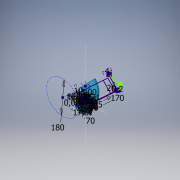
# Autodesk Inventor part: DriveChainEnclosure V3
Saved by Autodesk Inventor 2019.1 (Build 231200000, 200)
## iProperties
Created: 2018-07-04
Part Number: DriveChainEnclosure V3
Material: Generisch
Document SubType Name: Modeling
Designer: JochenAlt
Density: 1 g/cm^3
Appearance: Vorgabe
Mass: 189.121 g
Surface Area: 1542.72 cm^2
Volume: 189.121 cm^3
Author: JochenAlt
Autodesk Inventor part; units mm, degrees
ref_plane "YZ Plane" through (0, 0, 0) normal (1, 0, 0) x (0, 1, 0)
sketch "Enclosure" plane through (0, 0, 0) normal (0, 1, 0) x (-1, 0, 0)
  line L0 (35, 0) -> (-35, 0) construction
  circle A0 centre (26.215, 0) radius 8.785 construction
  circle A1 centre (-26.215, 0) radius 8.785 construction
  circle A2 centre (125, 0) radius 90 construction
  line L1 (0, -158.2918) -> (0, 319.751) construction
  line L2 (33.1583, 39.5344) -> (33.1583, 50.6343)
  line L3 (50.6835, 69.3012) -> (48.9666, 70.9023)
  line L4 (35, 0) -> (125, 0) construction
  line L5 (33.1583, 50.6343) -> (32.1474, 52.6444)
  arc A3 (33.1583, 50.6343) -> (33.3815, 50.747) centre (0, 116.5644) ccw
  line L6 (30.6583, 49.4353) -> (30.6583, 51.917)
  line L7 (33.3815, 50.747) -> (32.2506, 52.9767)
  line L8 (30.6583, 39.5344) -> (30.6583, 49.4353)
  line L9 (32.035, 52.8678) -> (30.9118, 55.1012)
  arc A4 (16, 52.2253) -> (31.759, 58.3675) centre (0, 116.5644) ccw
  arc A5 (0, 47.7657) -> (30.9118, 55.1012) centre (0, 116.5644) ccw
  arc A6 (-30.9118, 55.1012) -> (0, 47.7657) centre (0, 116.5644) ccw
  line L10 (33.7963, 54.6342) -> (31.759, 58.3675)
  line L11 (18.3935, -4) -> (-18.3935, -4) construction
  line L12 (18.3935, 4) -> (-18.3935, 4) construction
  line L13 (30.4083, 49.3217) -> (30.4083, 52.0753)
  arc A7 (16, 47.0842) -> (30.4083, 52.0753) centre (0, 116.5644) ccw
  line L14 (-30.6583, 39.5344) -> (-30.6583, 49.4353)
  line L15 (-30.6583, 49.4353) -> (-30.6583, 51.917)
  line L16 (-33.1583, 50.6343) -> (-32.1474, 52.6444)
  line L17 (-32.035, 52.8678) -> (-30.9118, 55.1012)
  line L18 (-30.4083, 49.3217) -> (-30.4083, 52.0753)
  arc A8 (-31.759, 58.3675) -> (-16, 52.2253) centre (0, 116.5644) ccw
  line L19 (-16, 50.1663) -> (-16, 52.2253)
  arc A9 (-30.8936, 55.6522) -> (-16, 50.1663) centre (0, 116.5644) ccw
  arc A10 (16, 50.1663) -> (30.8936, 55.6522) centre (0, 116.5644) ccw
  line L20 (-16, 49.6521) -> (-16, 47.0842)
  line L21 (-31.759, 58.3675) -> (31.759, 58.3675) construction
  arc A11 (-33.3815, 50.747) -> (-33.1583, 50.6343) centre (0, 116.5644) ccw
  arc A12 (-32.035, 52.8678) -> (-30.4083, 52.0753) centre (0, 116.5644) ccw
  line L22 (-33.3815, 50.747) -> (-32.2506, 52.9767)
  arc A13 (30.4083, 52.0753) -> (32.035, 52.8678) centre (0, 116.5644) ccw
  line L23 (32.2506, 52.9767) -> (30.8936, 55.6522)
  line L24 (16, 47.0842) -> (16, 49.6521)
  line L25 (16, 50.1663) -> (16, 52.2253)
  arc A14 (30.4083, 49.3217) -> (33.1583, 50.6343) centre (0, 116.5644) ccw
  arc A15 (0, 42.7657) -> (30.4083, 49.3217) centre (0, 116.5644) ccw
  arc A16 (0, 45.2657) -> (16, 47.0842) centre (0, 116.5644) ccw
  arc A17 (-30.6583, 49.4353) -> (-30.4083, 49.3217) centre (0, 116.5644) ccw
  arc A18 (-30.4083, 49.3217) -> (0, 42.7657) centre (0, 116.5644) ccw
  arc A19 (-30.4083, 52.0753) -> (0, 45.2657) centre (0, 116.5644) ccw
  line L26 (-30.8936, 55.6522) -> (-32.2506, 52.9767)
  line L27 (-32.2506, 52.9767) -> (-39.4034, 59.6467)
  line L28 (-31.759, 58.3675) -> (-33.7731, 54.3964)
  line L29 (32.2506, 52.9767) -> (33.7963, 54.6342)
  line L30 (33.7963, 54.6342) -> (48.9666, 70.9023)
  line L31 (33.3815, 50.747) -> (50.6835, 69.3012)
  line L32 (50.6835, 69.3012) -> (48.9666, 70.9023)
  line L33 (59.1782, 61.3799) -> (125, 0) construction
  line L34 (125, 0) -> (0, 116.5644) construction
  arc A20 (32.035, 52.8678) -> (32.2506, 52.9767) centre (0, 116.5644) ccw
  line L35 (0, 42.7657) -> (0, 45.2657)
  line L36 (0, 47.7657) -> (0, 45.2657)
  arc A21 (-32.2506, 52.9767) -> (-32.035, 52.8678) centre (0, 116.5644) ccw
  line L37 (16, 49.6521) -> (16, 50.1663)
  line L38 (-16, 49.6521) -> (-16, 50.1663)
  line L39 (-178.3606, 189.2264) -> (-131.6437, 239.3241) construction
  arc A22 (-33.1583, 50.6343) -> (-30.6583, 49.4353) centre (0, 116.5644) ccw
  line L40 (-41.1083, 57.8183) -> (-39.4034, 59.6467)
  line L41 (-39.4034, 59.6467) -> (-138.1361, 151.7165)
  arc A23 (-33.1583, 39.5344) -> (-35.3024, 49.664) centre (-58.1583, 39.5344) ccw
  line L42 (-33.1583, 50.6343) -> (-35.3024, 49.664)
  line L43 (-33.3815, 50.747) -> (-35.382, 49.8417)
  arc A24 (-35.382, 49.8417) -> (-41.1083, 57.8183) centre (-58.1583, 39.5344) ccw
  line L44 (42.1466, 63.5888) -> (0.4936, 102.4309)
  line L45 (0.4936, 102.4309) -> (-39.4034, 59.6467)
  line L46 (0.4936, 102.4309) -> (-123.8366, 218.3706)
  arc A25 (-35.3024, 49.664) -> (-35.382, 49.8417) centre (-58.1583, 39.5344) ccw
  line L47 (-138.1361, 151.7165) -> (-139.8411, 149.8881)
  line L48 (-123.8366, 218.3706) -> (-163.7335, 175.5864)
  line L49 (-138.1361, 151.7165) -> (-178.3606, 189.2264)
  line L50 (-41.1083, 57.8183) -> (-139.8411, 149.8881)
  line L51 (-180.0655, 187.398) -> (-139.8411, 149.8881)
  line L52 (-33.1583, 39.5344) -> (-30.6583, 39.5344) construction
  line L53 (-26, 14.7657) -> (-24.5156, 16.7773) construction
  spline S0 degree 4 poles (-33.1583, 39.5344) (-33.1583, 29.5735) (-31.4502, 7.8306) (0, 7.8211) (31.4502, 7.8306) (33.1583, 29.5735) (33.1583, 39.5344) knots 0 0 0 0 0 0.375 0.625 1 1 1 1 1
  line L54 (24.5156, 16.7773) -> (26, 14.7657) construction
  spline S1 degree 4 poles (-30.6583, 39.5344) (-30.6583, 30.3799) (-29.8014, 10.1412) (0, 10.5514) (29.8014, 10.1412) (30.6583, 30.3799) (30.6583, 39.5344) knots 0 0 0 0 0 0.375 0.625 1 1 1 1 1
  line L55 (-138.1361, 151.7165) -> (-98.2392, 194.5006)
  line L56 (-178.3606, 189.2264) -> (-180.0655, 187.398)
  spline S2 degree 3 poles (-180.0655, 187.398) (-233.1049, 241.3232) (-158.3203, 210.7169) (-131.6437, 239.3241) knots 0 0 0 0 1 1 1 1
  line L57 (-131.6437, 239.3241) -> (-128.7183, 236.5961)
  line L58 (-128.7183, 236.5961) -> (-175.4351, 186.4984)
  arc A26 (-30.6583, 48.886) -> (30.6583, 48.886) centre (0, 116.5644) ccw
  arc A27 (-32.1474, 52.6444) -> (-30.6583, 51.917) centre (0, 116.5644) ccw
  arc A28 (30.6583, 51.917) -> (32.1474, 52.6444) centre (0, 116.5644) ccw
  line L59 (-175.2987, 186.6446) -> (-178.2242, 189.3726)
  line L60 (-178.2242, 189.3726) -> (-178.3606, 189.2264)
  point P0 (0, 0)
  point P1 (0, 5)
  point P2 (0, 58.3675)
  point P3 (0, 8)
  point P4 (0, 22.5)
  point P5 (0, 10.5)
  point P6 (-191.4493, 221.539)
  point P7 (0, 50)
  dimension "d31" = 70
  dimension "d32" = 17.57
  dimension "d42" = 180
  dimension "d106" = 0
  dimension "d672" = 0.25
  dimension "d1173" = 2.5
  dimension "d1238" = 8
  dimension "d1249" = 0.25
  dimension "d1648" = 1
  dimension "d1792" = 32
  dimension "d1795" = 2
  dimension "d1872" = 10
  dimension "d2014" = 10
  dimension "d2069" = 135
  dimension "d2070" = 20
  dimension "d2071" = 2.5
  dimension "d2072" = 71
  dimension "d2075" = 170
  dimension "d2076" = 26
  dimension "d2077" = 28
  dimension "d2079" = 8
  dimension "d2080" = 14.5
  dimension "d2081" = 2.5
  dimension "d2082" = 3
  dimension "d2252" = 0.5
  dimension "d2255" = 0.25
  dimension "d2303" = 0.5
  dimension "d2367" = 2.5
  dimension "d2369" = 0.2
  dimension "d2370" = 4
  dimension "d2395" = 43
  dimension "d2396" = 50
  dimension "d2397" = 2.5
  dimension "d2398" = 25
  constraints: 124 end point, 79 point on circle, 29 centre point, 22 point on line, 16 perpendicular, 14 coincident, 12 vertical, 11 collinear, 9 parallel, 8 line through centre, 6 equal length, 5 horizontal alignment, 4 horizontal, 3 concentric, 3 equal radius, 2 midpoint, 2 tangent, 25 other
  measures "d31" distance of L0.end L0.start
  measures "d32" diameter of A0
  measures "d42" diameter of A2
  measures "d106" distance between parallel lines of L4 L0
  measures "d672" distance of L7.start L2.end
  measures "d1173" radial gap between concentric circles of A4 A5
  measures "d1238" distance between parallel lines of L11 L12
  measures "d1249" distance between parallel lines of L6 L13
  measures "d1648" distance from line of L12 point (0, 5)
  measures "d1792" distance between parallel lines of L25 L19
  measures "d1795" distance between parallel lines of L28 L26
  measures "d1872" distance from line of A3.centre L40
  measures "d2014" distance between parallel lines of L34 L44
  measures "d2069" distance between parallel lines of L45 L47
  measures "d2070" distance between parallel lines of L48 L39
  measures "d2071" distance of L40.start L27.end
  measures "d2072" distance between parallel lines of L50 L34
  measures "d2075" distance between parallel lines of L48 L45
  measures "d2077" vertical distance of L35.start L53.start
  measures "d2079" distance from line of point (0, 8) L0
  measures "d2080" distance of point (0, 22.5) point (0, 8)
  measures "d2081" distance of point (0, 10.5) point (0, 8)
  measures "d2082" distance of point (0, 5) point (0, 8)
  measures "d2252" radial gap between concentric circles of A10 A5
  measures "d2255" radial gap between concentric circles of A13 A28
  measures "d2303" radial gap between concentric circles of A15 A26
  measures "d2367" radial gap between concentric circles of A6 A19
  measures "d2369" distance between parallel lines of L49 L59
  measures "d2370" distance of L39.end L57.end
  measures "d2395" angle to the sketch y axis of L45
  measures "d2396" distance of point (0, 0) point (0, 50)
  measures "d2397" distance of L52.start L14.start
  measures "d2398" radius of A23
revolve "Umdrehung1" add sketch "Enclosure" angle 93 about axis through (-125, 0, 0) along (0.7313537, 0, 0.6819984) and the other way 27 contours S0 A23 L42 A22 L14 S1 L8 A14 L2 | A25 L43 A11 L42
ref_plane "Arbeitsebene52" through (0, 0, 5) normal (0, 0, 1) x (1, 0, 0)
sketch "OmniwheelBearing" plane through (0, 0, 5) normal (0, 0, 1) x (1, 0, 0)
  circle A0 centre (0, 0) radius 4.15
  circle A1 centre (0, 0) radius 5.65
  circle A2 centre (0, 0) radius 3.65
  line L0 (-91.936, 0) -> (21.9143, 0) construction
  line L1 (0, -28.1815) -> (0, 129.5388) construction
  dimension "d26" = 8.3
  dimension "d27" = 1.5
  dimension "d28" = 0.5
  constraints: 3 centre point, 2 coincident
  measures "d26" diameter of A0
  measures "d27" radial gap between concentric circles of A1 A0
  measures "d28" radial gap between concentric circles of A0 A2
extrude "Extrusion254" add sketch "OmniwheelBearing" along normal up to next contours A1
chamfer "Fase24" distance 3 angle 45 2 edges at (3.6916, -4.2772, 8.1473) (-3.6918, 4.2771, 8.1472)
extrude "Extrusion258" cut sketch "OmniwheelBearing" along normal through all contours A0 | A1 | A2
extrude "Extrusion264" add sketch "OmniwheelBearing" along normal blind 6 contours A0 | A1
extrude "Extrusion265" add sketch "OmniwheelBearing" along normal blind 3 from surface at 6 contours A1
ref_plane "Arbeitsebene88" through (0, 0, 22.5) normal (0, 0, 1) x (1, 0, 0)
sketch "PlanetaryHolder" plane through (0, 0, 22.5) normal (0, 0, 1) x (1, 0, 0)
  circle A0 centre (0, 0) radius 28.7
  arc A1 (11.2121, 24.2318) -> (9.2063, 25.0626) centre (10.1411, 24.4828) ccw
  arc A2 (9.2063, -25.0626) -> (11.2121, -24.2318) centre (10.1411, -24.4828) ccw
  arc A3 (-24.2318, 11.2121) -> (-25.0626, 9.2063) centre (-24.4828, 10.1411) ccw
  arc A4 (24.2318, -11.2121) -> (25.0626, -9.2063) centre (24.4828, -10.1411) ccw
  arc A5 (25.0626, 9.2063) -> (24.2318, 11.2121) centre (24.4828, 10.1411) ccw
  arc A6 (-11.2121, -24.2318) -> (-9.2063, -25.0626) centre (-10.1411, -24.4828) ccw
  arc A7 (-25.0626, -9.2063) -> (-24.2318, -11.2121) centre (-24.4828, -10.1411) ccw
  arc A8 (-9.2063, 25.0626) -> (-11.2121, 24.2318) centre (-10.1411, 24.4828) ccw
  arc A9 (24.2318, 11.2121) -> (11.2121, 24.2318) centre (0, 0) ccw
  arc A10 (25.0626, -9.2063) -> (25.0626, 9.2063) centre (0, 0) ccw
  arc A11 (11.2121, -24.2318) -> (24.2318, -11.2121) centre (0, 0) ccw
  arc A12 (-24.2318, -11.2121) -> (-11.2121, -24.2318) centre (0, 0) ccw
  arc A13 (9.2063, 25.0626) -> (-9.2063, 25.0626) centre (0, 0) ccw
  arc A14 (24.2318, 11.2121) -> (11.2121, 24.2318) centre (0, 0) ccw
  arc A15 (9.2063, 25.0626) -> (-9.2063, 25.0626) centre (0, 0) ccw
  arc A16 (-11.2121, 24.2318) -> (-24.2318, 11.2121) centre (0, 0) ccw
  arc A17 (-11.2121, 24.2318) -> (-24.2318, 11.2121) centre (0, 0) ccw
  arc A18 (-25.0626, 9.2063) -> (-25.0626, -9.2063) centre (0, 0) ccw
  arc A19 (-25.0626, 9.2063) -> (-25.0626, -9.2063) centre (0, 0) ccw
  arc A20 (-24.2318, -11.2121) -> (-11.2121, -24.2318) centre (0, 0) ccw
  arc A21 (-9.2063, -25.0626) -> (9.2063, -25.0626) centre (0, 0) ccw
  arc A22 (-9.2063, -25.0626) -> (9.2063, -25.0626) centre (0, 0) ccw
  arc A23 (11.2121, -24.2318) -> (24.2318, -11.2121) centre (0, 0) ccw
  arc A24 (25.0626, -9.2063) -> (25.0626, 9.2063) centre (0, 0) ccw
  line L0 (-24.4828, 10.1411) -> (24.4828, -10.1411) construction
  line L1 (10.1411, -24.4828) -> (-10.1411, 24.4828) construction
  line L2 (24.4828, 10.1411) -> (-24.4828, -10.1411) construction
  line L3 (10.1411, 24.4828) -> (-10.1411, -24.4828) construction
  line L4 (0, 137.5768) -> (0, -76.4098) construction
  line L5 (0, -76.4098) -> (0, 137.5768) construction
  circle A25 centre (0, 0) radius 26.2
  circle A26 centre (0, 0) radius 26.5 construction
  circle A27 centre (22.3013, 23.9153) radius 1.25
  circle A28 centre (22.3013, -23.9153) radius 1.25
  circle A29 centre (-22.3013, -23.9153) radius 1.25
  circle A30 centre (-22.3013, 23.9153) radius 1.25
  arc A31 (19.6956, 22.4287) -> (19.6956, 22.4287) centre (22.3013, 23.9153) ccw
  line L6 (24.4954, -21.8693) -> (21.6602, -18.8289)
  line L7 (17.2721, -22.9209) -> (20.1073, -25.9613)
  arc A32 (20.1073, -25.9613) -> (24.4954, -21.8693) centre (22.3013, -23.9153) ccw
  circle A33 centre (22.3013, -23.9153) radius 2.5
  circle A34 centre (22.3013, 23.9153) radius 2.5
  arc A35 (24.4954, 21.8693) -> (20.1073, 25.9613) centre (22.3013, 23.9153) ccw
  line L8 (24.4954, 21.8693) -> (21.6602, 18.8289)
  line L9 (17.2721, 22.9209) -> (20.1073, 25.9613)
  circle A36 centre (-22.3013, 23.9153) radius 2.5
  arc A37 (-24.4954, -21.8693) -> (-20.1073, -25.9613) centre (-22.3013, -23.9153) ccw
  line L10 (-21.6602, 18.8289) -> (-24.4954, 21.8693)
  line L11 (-21.6602, -18.8289) -> (-24.4954, -21.8693)
  line L12 (-17.2721, -22.9209) -> (-20.1073, -25.9613)
  arc A38 (-20.1594, 26.0157) -> (-24.4954, 21.8693) centre (-22.3013, 23.9153) ccw
  circle A39 centre (-22.3013, -23.9153) radius 2.5
  arc A40 (20.1073, 25.9613) -> (24.4954, 21.8693) centre (22.3013, 23.9153) ccw
  circle A41 centre (0, 0) radius 32.7 construction
  arc A42 (20.1073, -25.9613) -> (24.4954, -21.8693) centre (22.3013, -23.9153) ccw
  line L13 (22.3013, -23.9153) -> (-22.3013, 23.9153) construction
  line L14 (22.3013, 23.9153) -> (-25.6845, -27.5432) construction
  arc A43 (24.4954, -21.8693) -> (20.1073, -25.9613) centre (22.3013, -23.9153) ccw
  arc A44 (-24.4954, 21.8693) -> (-20.1594, 26.0157) centre (-22.3013, 23.9153) ccw
  arc A45 (-20.2567, -26.1106) -> (-24.4954, -21.8693) centre (-22.3013, -23.9153) ccw
  line L15 (-17.2721, 22.9209) -> (-20.1073, 25.9613)
  point P0 (0, 0)
  point P1 (0, 0)
  point P2 (0, 0)
  point P3 (0, 0)
  dimension "d2393" = 26.5
  dimension "d2384" = 2.2
  dimension "d2387" = 2
  dimension "d2388" = 0.5
  dimension "d2394" = 0.2
  dimension "d2399" = 2.5
  dimension "d2407" = 5
  dimension "d2408" = 0.5
  dimension "d2430" = 45
  dimension "d2431" = 4
  dimension "d2432" = 94
  constraints: 77 point on circle, 44 centre point, 29 end point, 25 coincident, 24 equal radius, 12 tangent, 10 midpoint, 4 parallel, 4 point on line, 2 perpendicular, 26 other
  measures "d2384" diameter of A8
  measures "d2388" radial gap between concentric circles of A9 A25
  measures "d2399" diameter of A28
  measures "d2407" diameter of A33
  measures "d2408" radial gap between concentric circles of A32 A33
  measures "d2430" angle of L1 L3
  measures "d2432" angle of L13 L14
extrude "Extrusion382" add sketch "PlanetaryHolder" against normal up to next contours A0 | A0 L9 A31 L8 | L6 A43 L7 A0 | A31 | A32 A43 | A0 L10 A44 L15 | L12 A45 L11 A0 | A44 A38 | A37 A45 | A28 | A33
extrude "Extrusion383" add sketch "PlanetaryHolder" along normal blind 8 contours A0 | A0 L9 A31 L8 | L6 A43 L7 A0 | A31 | A32 A43 | A0 L10 A44 L15 | L12 A45 L11 A0 | A44 A38 | A37 A45 | A33 | A34 | A36 | A39
extrude "Extrusion384" cut sketch "PlanetaryHolder" against normal through all contours A27 | A28 | A29 | A30 | A33 | A34 | A36 | A39
extrude "Extrusion385" add sketch "PlanetaryHolder" along normal blind 13 from surface at 8 separate body contours A31 | A32 A43 | A44 A38 | A37 A45 | A33 | A34 | A36 | A39
sketch "MotorConnector" plane through (22.5292, 23.9153, 43.5) normal (0, 0, 1) x (1, 0, 0)
  circle A0 centre (-0.2279, 0) radius 3 projected
  circle A1 centre (-0.2279, 0) radius 1.25 projected
  circle A2 centre (-0.2279, -47.8305) radius 1.25 projected
  circle A3 centre (-44.8306, -47.8305) radius 3 projected
  circle A4 centre (-44.8306, -47.8305) radius 1.25 projected
  circle A5 centre (-44.8306, 0) radius 1.25 projected
  circle A6 centre (-44.8306, 0) radius 3 projected
  circle A7 centre (-22.5292, -23.9153) radius 15.25
  arc A8 (-4.9562, -21.4153) -> (-4.9562, -26.4153) centre (-22.5292, -23.9153) ccw
  line L0 (1.9662, -2.046) -> (-8.4038, -13.1665)
  line L1 (-2.4219, 2.046) -> (-12.792, -9.0745)
  line L2 (1.9662, -45.7845) -> (-8.4038, -34.664)
  line L3 (-12.792, -38.756) -> (-2.4219, -49.8765)
  line L4 (-36.6546, -34.664) -> (-47.0246, -45.7845)
  line L5 (-32.2665, -38.756) -> (-42.6365, -49.8765)
  circle A9 centre (-44.8306, 0) radius 3 construction
  circle A10 centre (-44.8306, -47.8305) radius 3 construction
  line L6 (-32.2665, -9.0745) -> (-42.6365, 2.046)
  line L7 (-36.6546, -13.1665) -> (-47.0246, -2.046)
  arc A11 (-42.6365, 2.046) -> (-47.0246, -2.046) centre (-44.8306, 0) ccw
  line L8 (-44.1894, -42.7441) -> (-47.0246, -45.7845) projected
  arc A12 (-47.0246, -45.7845) -> (-42.6365, -49.8765) centre (-44.8306, -47.8305) ccw
  line L9 (-10.1379, -15.0261) -> (-8.4038, -13.1665)
  line L10 (-10.1379, -32.8045) -> (-8.4038, -34.664)
  line L11 (-10.5533, -10.8142) -> (1.0438, -21.4153)
  line L12 (1.0438, -21.4153) -> (1.0438, -23.4153)
  line L13 (1.0438, -26.4153) -> (-10.5533, -37.0164)
  line L14 (1.0438, -23.4153) -> (-4.7863, -23.4153)
  line L15 (-7.2874, -24.4153) -> (-4.7863, -24.4153)
  line L16 (-23.0228, -23.9153) -> (101.3074, -23.9153) construction
  line L17 (1.0438, -26.4153) -> (-4.9562, -26.4153)
  line L18 (1.0438, -21.4153) -> (-4.9562, -21.4153)
  arc A13 (-4.7863, -23.4153) -> (-4.9562, -21.4153) centre (-22.5292, -23.9153) ccw
  line L19 (-4.7863, -23.4153) -> (-7.2874, -23.4153)
  line L20 (1.0438, -23.4153) -> (1.0438, -24.4153)
  line L21 (1.0438, -24.4153) -> (1.0438, -26.4153)
  arc A14 (-4.7863, -24.4153) -> (-4.7863, -23.4153) centre (-22.5292, -23.9153) ccw
  arc A15 (-4.9562, -26.4153) -> (-4.7863, -24.4153) centre (-22.5292, -23.9153) ccw
  line L22 (-4.7863, -24.4153) -> (1.0438, -24.4153)
  arc A16 (-2.4219, -49.8765) -> (1.9662, -45.7845) centre (-0.2279, -47.8305) ccw
  line L23 (-0.2279, -47.8305) -> (-44.8306, 0) construction
  line L24 (-0.2279, 0) -> (-44.8306, -47.8305) construction
  arc A17 (1.9662, -2.046) -> (-2.4219, 2.046) centre (-0.2279, 0) ccw
  circle A18 centre (-0.2279, -47.8305) radius 3 construction
  dimension "d2419" = 1
  dimension "d2420" = 2
  dimension "d2421" = 6
  dimension "d2433" = 30.5
  dimension "d2434" = 2.5
  constraints: 46 end point, 14 point on circle, 11 tangent, 6 centre point, 6 coincident, 5 collinear, 5 parallel, 2 point on line, 65 other
  measures "d2419" distance between parallel lines of L15 L14
  measures "d2420" distance between parallel lines of L17 L15
  measures "d2421" distance of L13.start L17.end
  measures "d2433" diameter of A7
extrude "Extrusion386" add sketch "MotorConnector" along normal blind 3 contours A0 | A0 L0 L11 A8 L1 | A8 L9 A7 L10 | L0 A8 L11 | A8 L7 A6 L6 | A6 | A8 L5 A3 L4 | L2 L13 A8 | A8 L13 L2 A16 L3 | A3 bodies 2
extrude "Extrusion387" add sketch "MotorConnector" along normal blind 6 from surface at 3 contours A8 L9 A7 L10 bodies 2
extrude "Extrusion388" add sketch "MotorConnector" along normal blind 15 from surface at 9 contours A8 L9 A7 L10 | L11 L18 A8 L0 | L0 A8 L11 | A8 A13 L19 A7 L9 | L12 L14 A13 L18 | A7 L15 A15 A8 L10 | L21 L17 A15 L22 | L2 L13 A8 | A8 L17 L13 L2 bodies 2
ref_plane "Arbeitsebene89" through (15.2418, 0, 67.5) normal (0, -1, 0) x (1, 0, 0)
sketch "Skizze102" plane through (15.2418, 0, 67.5) normal (0, -1, 0) x (1, 0, 0)
  line L0 (8.3313, 0) -> (0, 0) construction
  line L1 (0, -15) -> (0, 0) construction
  line L2 (8.3313, -15) -> (0, -15) construction
  line L3 (8.3313, 0) -> (8.3313, -15) construction
  line L4 (0, -7.5) -> (8.3313, -7.5) construction
  line L5 (8.3313, 0) -> (8.3313, -15) construction
  circle A0 centre (4.1656, -7.5) radius 1.25
  circle A1 centre (4.1656, -7.5) radius 3
  line L6 (4.1656, -4.5) -> (8.3313, -4.5)
  line L7 (8.3313, -4.5) -> (8.3313, -10.5)
  line L8 (8.3313, -10.5) -> (4.1656, -10.5)
  point P0 (-15.2418, -67.5)
  dimension "d2422" = 2.5
  dimension "d2423" = 6
  dimension "d1205" = 2.4
  dimension "d1209" = 8
  dimension "d1216" = 5
  dimension "d1618" = 0.4
  dimension "d1701" = 38
  dimension "d1774" = 0.2
  dimension "d1775" = 40
  dimension "d1776" = 2
  dimension "d2327" = 46
  dimension "d2328" = 45
  dimension "d2329" = 0.5
  dimension "d891" = 43.57
  dimension "d892" = 6.6
  dimension "d893" = 31.3
  dimension "d1081" = 8.2
  dimension "d1082" = 1.5
  dimension "d1087" = 1
  dimension "d1625" = 99.6
  dimension "d1749" = 1
  dimension "d1750" = 17.1
  dimension "d1716" = 30.4
  dimension "d1717" = 2
  dimension "d1718" = 2
  dimension "d1719" = 7
  dimension "d1720" = 7
  dimension "d1784" = 0.5
  dimension "d1737" = 2.5
  dimension "d1738" = 8
  dimension "d1739" = 6
  dimension "d1740" = 3
  constraints: 8 end point, 4 midpoint, 2 centre point, 2 point on circle, 2 point on line, 2 tangent, 1 coincident, 1 horizontal, 1 parallel, 1 other
  measures "d2422" diameter of A0
  measures "d2423" diameter of A1
extrude "Extrusion389" add sketch "Skizze102" along normal through all both and the other way through all separate body contours A0 | A1 | A1 L6 L7 L8
extrude "Extrusion390" cut sketch "Skizze102" along normal mid plane 5 bodies 3
combine bodies "Kombinieren71" operation type subtract main body 2 bodies to subtract 3
sketch "Skizze81" plane through (0, 0, 0) normal (0, 0, 1) x (1, 0, 0)
  ellipse E0 centre (-43.5519, 0) end of major axis (-43.5519, 38.9643) minor radius 27.5519 (-16.379, 6.441) -> (-17.9382, 13.9202) ccw construction
  ellipse E1 centre (-27.5519, 0) end of major axis (-27.5519, -61.5917) minor radius 43.5519 (15.621, 8.1084) -> (14.8292, 13.9202) ccw construction
  line L0 (14.8743, 13.928) -> (14.5198, 15.9899)
  line L1 (-17.8213, 13.9538) -> (-18.3922, 15.9384)
  line L2 (-17.9382, 13.9202) -> (14.8292, 13.9202)
  ellipse E2 centre (-5.2199, 30.8617) end of major axis (-7.5919, 44.6593) minor radius 20 (14.491, 34.2503) -> (-24.9307, 27.4731) ccw
  line L3 (-7.5919, 44.6593) -> (-0.424, 2.9651) construction
  line L4 (-5.2199, 30.8617) -> (14.491, 34.2503) construction
  arc A0 (14.5198, 15.9899) -> (14.491, 34.2503) centre (-39.1097, 25.0355) ccw
  line L5 (-5.2199, 30.8617) -> (-24.9307, 27.4731) construction
  arc A1 (-24.9307, 27.4731) -> (-18.3922, 15.9384) centre (-5.6352, 30.7903) ccw
  point P0 (0, 0)
  dimension "d1909" = 20
  dimension "d1910" = 14
  dimension "d1912" = 2.1
  dimension "d1913" = 2.1
  dimension "d1875" = 2.4
  dimension "d1876" = 2
  dimension "d1879" = 5
  dimension "d2001" = 12
  dimension "d2006" = 25
  dimension "d2219" = 3
  dimension "d1832" = 50
  dimension "d1871" = 21
  dimension "d1903" = 12
  dimension "d1904" = 2
  dimension "d1918" = 15.3
  dimension "d1928" = 6
  dimension "d1929" = 24
  dimension "d1984" = 6
  dimension "d2024" = 9
  dimension "d2025" = 45
  dimension "d2026" = 16.5
  dimension "d2027" = 30
  dimension "d2029" = 35
  dimension "d2030" = 2.5
  dimension "d2046" = 2.5
  dimension "d2309" = 4.4
  dimension "d2325" = 1
  dimension "d2360" = 18
  dimension "d2363" = 134
  dimension "d2368" = 54
  dimension "d2351" = 16
  dimension "d1958" = 6.2
  dimension "d1959" = 1
  dimension "d1960" = 1.5
  dimension "d2009" = 4
  dimension "d2041" = 14.7
  dimension "d2045" = 14
  dimension "d2178" = 14
  dimension "d2204" = 10.5
  dimension "d2225" = 1
  dimension "d2243" = 27
  dimension "d2350" = 4.25
  dimension "d2366" = 120
  dimension "d2057" = 3.2
  dimension "d2140" = 1.5
  dimension "d2142" = 63
  dimension "d2143" = 3.5
  dimension "d2150" = 66.7
  dimension "d2151" = 4
  dimension "d2230" = 60
  dimension "d2331" = 0.3
  dimension "d2359" = 0.3
  dimension "d2232" = 6.2
  dimension "d2233" = 1
  dimension "d2239" = 30
  dimension "d2241" = 10
  dimension "d2277" = 19
  dimension "d2278" = 12.5
  dimension "d2279" = 2.5
  dimension "d2280" = 5
  dimension "d2281" = 2.5
  dimension "d2283" = 6
  dimension "d2285" = 35
  dimension "d2299" = 5
  constraints: 22 end point, 5 parallel, 4 collinear, 4 midpoint, 4 perpendicular, 2 point on circle, 1 centre point, 1 line through centre, 2 other
  measures "d2279" distance between parallel lines of L1 L3
  measures "d2280" diameter of A0
  measures "d2283" distance from line of point (243.5, 70.903) L5
  measures "d2285" distance of L2.end L3.end
sketch "Skizze90" plane through (-48.4368, 0, 76.5632) normal (0.7071068, 0, 0.7071068) x (-0.3438236, -0.8738253, 0.3438236)
  line L0 (-7.418, 3.1009) -> (9.2853, 3.1009) construction
  line L1 (9.2853, 3.1009) -> (9.2853, -5.6766) construction
  line L2 (9.2853, -5.6766) -> (-7.418, -5.6766) construction
  line L3 (-7.418, -5.6766) -> (-7.418, 3.1009) construction
  line L4 (27.8783, 2.2736) -> (27.8783, -2.3039) construction
  line L5 (27.8783, -2.3039) -> (21.7585, -2.3039) construction
  line L6 (21.7585, -2.3039) -> (21.7585, 2.2736) construction
  line L7 (21.7585, 2.2736) -> (27.8783, 2.2736) construction
  line L8 (-8.4972, -19.7227) -> (-4.5329, -22.0114) construction
  line L9 (-4.5329, -22.0114) -> (-7.6472, -27.4055) construction
  line L10 (-7.6472, -27.4055) -> (-11.6114, -25.1167) construction
  line L11 (-11.6114, -25.1167) -> (-8.4972, -19.7227) construction
  line L12 (-16.6865, 22.6495) -> (-12.7223, 24.9383) construction
  line L13 (-12.7223, 24.9383) -> (-9.5437, 19.4329) construction
  line L14 (-9.5437, 19.4329) -> (-13.5079, 17.1442) construction
  line L15 (-13.5079, 17.1442) -> (-16.6865, 22.6495) construction
  arc A0 (2.7289, 27.8374) -> (-25.0941, 12.3553) centre (0, 0) ccw construction
  arc A1 (-25.2864, -11.9569) -> (2.2882, -27.8771) centre (0, 0) ccw construction
  arc A2 (2.2882, 27.8771) -> (-25.2864, 11.9569) centre (0, 0) ccw construction
  point P0 (-42.978, 77.236)
  point P1 (-9.6293, -26.2611)
  point P2 (-14.7044, 23.7939)
  constraints: 3 point on circle, 2 midpoint, 8 other
sketch "Skizze91" plane through (-5.2199, 30.8617, 57.3677) normal (0, 0, 1) x (0.9619333, 0.2732844, 0)
  line L0 (-6.1802, -3.2982) -> (0.5305, -3.2982) construction
  line L1 (0.5305, -3.2982) -> (0.5305, -6.9457) construction
  line L2 (0.5305, -6.9457) -> (-6.1802, -6.9457) construction
  line L3 (-6.1802, -6.9457) -> (-6.1802, -3.2982) construction
  point P0 (-3.4129, -31.1134)
  constraints: 2 other
sketch "Skizze94" plane through (-33, 0, 33.8894) normal (-1, 0, 0) x (0, -1, 0)
  line L0 (-4.5537, 18.5969) -> (7.1421, 18.5969) construction
  line L1 (7.1421, 18.5969) -> (7.1421, 12.2399) construction
  line L2 (7.1421, 12.2399) -> (-4.5537, 12.2399) construction
  line L3 (-4.5537, 12.2399) -> (-4.5537, 18.5969) construction
  point P0 (0, -33.8894)
  constraints: 2 other
equation "\"d851\" = 60deg"
equation "\"Skizze50_Pitch\" = 2.30909"
